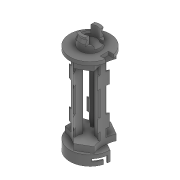
# Autodesk Inventor part: Sujección_Baterias
Saved by Autodesk Inventor 2022.3 (Build 263350000, 350)
## iProperties
Created: 2023-07-18
Part Number: Sujección_Baterias
Material: Genérico
Document SubType Name: Modeling
Designer: Usuario
Density: 1 g/cm^3
Appearance: Valor por defecto
Author: Usuario
Autodesk Inventor part; units mm, degrees
ref_plane "YZ Plane" through (0, 0, 0) normal (1, 0, 0) x (0, 1, 0)
ref_plane "XZ Plane" through (0, 0, 0) normal (0, 1, 0) x (-1, 0, 0)
ref_plane "XY Plane" through (0, 0, 0) normal (0, 0, 1) x (1, 0, 0)
sketch "Boceto1" plane through (0, 0, 0) normal (0, 1, 0) x (-1, 0, 0)
  circle A0 centre (0, 0) radius 10.5
  circle A1 centre (0, 0) radius 7.25
  dimension "d0" = 21
  dimension "d1" = 14.5
  constraints: 2 centre point, 2 coincident
  measures "d0" diameter of A0
  measures "d1" diameter of A1
extrude "Extrusión1" add sketch "Boceto1" along normal blind 14
sketch "Boceto2" plane through (0, 14, 0) normal (0, 1, 0) x (1, 0, 0)
  line L0 (0, 0) -> (-4.6, 0)
  line L1 (-4.6, 0) -> (-4.6, -9.4387)
  circle A0 centre (0, 0) radius 10.5 projected
  line L2 (-4.6, 0) -> (-4.6, 9.4387)
  line L3 (0, 0) -> (4.6, 0)
  line L4 (4.6, 0) -> (4.6, -9.4387)
  line L5 (4.6, 0) -> (4.6, 9.4387)
  circle A1 centre (0, 0) radius 10.5
  dimension "d4" = 4.6
  dimension "d5" = 4.6
  constraints: 12 end point, 4 point on circle, 3 point on line, 2 perpendicular, 1 centre point, 1 coincident, 1 horizontal
  measures "d4" distance of L0.start L0.end
  measures "d5" distance of L3.start L3.end
extrude "Extrusión2" cut sketch "Boceto2" against normal blind 8 contours L1 A0 L2 | L5 A0 L4
sketch "Boceto3" plane through (0, 6, 0) normal (0, 1, 0) x (1, 0, 0)
  arc A0 (4.6, -9.4387) -> (4.6, 9.4387) centre (0, 0) ccw projected
  line L0 (10.5, 0) -> (7.25, 0)
  circle A1 centre (0, 0) radius 7.25 projected
  line L1 (8.875, 0) -> (8.875, -5)
  line L2 (8.875, -5) -> (5.25, -5)
  line L3 (8.875, 0) -> (8.875, 5)
  line L4 (8.875, 5) -> (5.25, 5)
  line L5 (8.875, -5) -> (9.2331, -5)
  line L6 (8.875, 5) -> (9.2331, 5)
  arc A2 (4.6, -5.6038) -> (4.6, 5.6038) centre (0, 0) ccw projected
  dimension "d8" = 5
  dimension "d9" = 5
  constraints: 14 end point, 6 point on circle, 3 perpendicular, 2 vertical, 1 horizontal, 1 midpoint, 1 parallel
  measures "d8" distance of L1.start L1.end
  measures "d9" distance of L1.start L3.end
extrude "Extrusión3" cut sketch "Boceto3" against normal blind 3 contours L5 L1 L0 A0 | L0 L3 L6 A0 | L2 A1 L0 L1 | L0 A1 L4 L3
sketch "Boceto4" plane through (0, 0, 0) normal (1, 0, 0) x (0, 1, 0)
  line L0 (14, 9.4387) -> (14, 10.5) projected
  line L1 (14, 5.6038) -> (6, 5.6038) projected
  line L2 (7.5, 8.75) -> (14, 8.75)
  line L3 (14, 12.25) -> (7.5, 12.25)
  line L4 (7.5, 12.25) -> (7.5, 8.75)
  line L5 (7.5, 10.5) -> (10.75, 8.75)
  line L6 (10.75, 8.75) -> (14, 10.5)
  line L7 (14, 10.5) -> (14, 12.25)
  line L8 (14, 10.5) -> (14, 8.75)
  line L9 (14, 8.75) -> (7.5, 8.75)
  line L10 (7.5, 8.75) -> (7.5, 10.5)
  point P0 (0, 0)
  constraints: 18 end point, 3 perpendicular, 2 midpoint, 1 parallel
sketch3d "Boceto 3D1"
  arc A0 (-10.5, 0, 0) -> (0, 0, 10.5) centre (0, 0, 0) ccw
  arc A1 (0, 0, 10.5) -> (10.5, 0, 0) centre (0, 0, 0) ccw
  arc A2 (10.5, 0, 0) -> (0, 0, -10.5) centre (0, 0, 0) ccw
  arc A3 (0, 0, -10.5) -> (-10.5, 0, 0) centre (0, 0, 0) ccw
sweep "Barrido1" cut profiles "Boceto4" path "Boceto 3D1" contours L6 L5 L4 L3 L7
sketch "Boceto6" plane through (0, 3, 0) normal (0, 1, 0) x (1, 0, 0)
  circle A0 centre (0, 0) radius 7.25
  constraints: 1 centre point, 1 coincident
extrude "Extrusión4" add sketch "Boceto6" against normal blind 3
sketch "Boceto5" plane through (0, 0, 0) normal (0, -1, 0) x (1, 0, 0)
  circle A0 centre (0, 0) radius 21
  dimension "d16" = 42
  constraints: 1 centre point, 1 coincident
  measures "d16" diameter of A0
extrude "Extrusión5" add sketch "Boceto5" along normal blind 3.7
sketch "Boceto7" plane through (0, -3.7, 0) normal (0, -1, 0) x (1, 0, 0)
  circle A0 centre (0, 0) radius 21 projected
  line L0 (-21, 0) -> (15, 0)
  line L1 (15, 0) -> (15, 4.375)
  line L2 (15, 4.375) -> (20.5392, 4.375)
  line L3 (15, 0) -> (15, -4.375)
  line L4 (15, -4.375) -> (20.5392, -4.375)
  circle A1 centre (0, 0) radius 21 projected
  dimension "d19" = 36
  dimension "d20" = 4.375
  dimension "d21" = 4.375
  constraints: 10 end point, 3 point on circle, 1 horizontal, 1 perpendicular, 1 point on line, 1 vertical
  measures "d19" distance of L0.start L0.end
  measures "d20" distance of L0.end L1.end
  measures "d21" distance of L0.end L3.end
extrude "Extrusión6" cut sketch "Boceto7" against normal through all contours A0 L4 L3 L1 L2
sketch "Boceto8" plane through (0, -3.7, 0) normal (0, -1, 0) x (1, 0, 0)
  arc A0 (4.6, 9.4387) -> (-4.6, 9.4387) centre (0, 0) ccw projected
  arc A1 (20.5392, 4.375) -> (20.5392, -4.375) centre (0, 0) ccw projected
  line L0 (-21, 0) -> (10.5, 18.1865)
  line L1 (10.5, 18.1865) -> (10.5, -18.1865)
  line L2 (10.5, -18.1865) -> (-21, 0)
  line L3 (10.5, 18.1865) -> (0, 0)
  line L4 (0, 0) -> (10.5, -18.1865)
  line L5 (0, 0) -> (-21, 0)
  line L6 (10.5, 18.1865) -> (6, 10.3923)
  line L7 (10.5, -18.1865) -> (6, -10.3923)
  line L8 (-21, 0) -> (-12, 0)
  circle A2 centre (-12, 0) radius 9
  circle A3 centre (6, -10.3923) radius 9
  circle A4 centre (6, 10.3923) radius 9
  line L9 (0, 0) -> (-22.5, 38.9711)
  circle A5 centre (-22.5, 38.9711) radius 31.3609
  line L10 (0, 0) -> (-22.5, -38.9711)
  line L11 (0, 0) -> (45, 0)
  circle A6 centre (-22.5, -38.9711) radius 31.3609
  circle A7 centre (45, 0) radius 31.3609
  line L12 (10.5, 18.1865) -> (9, 15.5885)
  line L13 (9, 15.5885) -> (2.1283, 19.5559)
  line L14 (9, 15.5885) -> (15.8717, 11.6211)
  line L15 (-21, 0) -> (-18, 0)
  line L16 (-18, 0) -> (-18, 7.9348)
  line L17 (-18, 0) -> (-18, -7.9348)
  line L18 (10.5, -18.1865) -> (9, -15.5885)
  line L19 (9, -15.5885) -> (15.8717, -11.6211)
  line L20 (9, -15.5885) -> (2.1283, -19.5559)
  dimension "d24" = 9
  dimension "d25" = 9
  dimension "d26" = 45
  dimension "d27" = 45
  dimension "d28" = 45
  dimension "d29" = 3
  dimension "d30" = 3
  dimension "d31" = 3
  constraints: 42 end point, 8 point on line, 7 coincident, 7 point on circle, 3 centre point, 3 perpendicular, 2 horizontal, 1 horizontal alignment, 18 other
  measures "d24" distance of L0.end L6.end
  measures "d25" distance of L0.start L8.end
  measures "d26" distance of L3.end L9.end
  measures "d27" distance of L3.end L10.end
  measures "d28" distance of L3.end L11.end
  measures "d29" distance of L0.end L12.end
  measures "d30" distance of L0.start L15.end
  measures "d31" distance of L1.end L18.end
extrude "Extrusión7" add sketch "Boceto8" along normal blind 6.3 contours A7 A4 L14 | L13 L3 A4 L0 | L0 A4 L13 | L14 A4 L1 | L1 A4 L3 L14 | A4 A5 L13 | A7 L11 L1 A4 | A4 L3 L9 L0 | L0 L9 A5 A4 | L1 L11 L3 A4 | L19 A3 A7 | A7 A3 L1 L11 | L9 L0 A2 A5 | L9 L5 A2 L0 | L1 A3 L4 L11 | L19 L4 A3 L1 | L1 A3 L19 | L20 A3 L2 | L2 A3 L4 L20 | L20 A6 A3 | A5 A2 L16 | A2 L0 L16 | A2 L5 L16 L0 | L10 L2 A2 L5 | L4 A3 L2 L10 | A3 A6 L10 L2 | L17 L5 A2 L2 | L2 A2 L17 | A2 A6 L17 | L10 A6 A2 L2 picked at (0.5579, 12.9993) picked at (10.9788, 6.9828) picked at (10.9788, -6.9828) picked at (0.5579, -12.9993) picked at (-11.5367, 6.0165) picked at (-11.5367, -6.0165)
sketch "Boceto9" plane through (0, -10, 0) normal (0, -1, 0) x (1, 0, 0)
  arc A0 (4.6, 9.4387) -> (-4.6, 9.4387) centre (0, 0) ccw
  arc A1 (20.5392, 4.375) -> (20.5392, -4.375) centre (0, 0) ccw
  line L0 (-21, 0) -> (10.5, 18.1865)
  line L1 (10.5, 18.1865) -> (10.5, -18.1865)
  line L2 (10.5, -18.1865) -> (-21, 0)
  line L3 (10.5, 18.1865) -> (0, 0)
  line L4 (0, 0) -> (10.5, -18.1865)
  line L5 (0, 0) -> (-21, 0)
  line L6 (10.5, 18.1865) -> (6, 10.3923)
  line L7 (10.5, -18.1865) -> (6, -10.3923)
  line L8 (-21, 0) -> (-12, 0)
  circle A2 centre (-12, 0) radius 9
  circle A3 centre (6, -10.3923) radius 9
  circle A4 centre (6, 10.3923) radius 9
  line L9 (0, 0) -> (-22.5, 38.9711)
  circle A5 centre (-22.5, 38.9711) radius 31.3609
  line L10 (0, 0) -> (-22.5, -38.9711)
  line L11 (0, 0) -> (45, 0)
  circle A6 centre (-22.5, -38.9711) radius 31.3609
  circle A7 centre (45, 0) radius 31.3609
  line L12 (10.5, 18.1865) -> (9, 15.5885)
  line L13 (9, 15.5885) -> (2.1283, 19.5559)
  line L14 (9, 15.5885) -> (15.8717, 11.6211)
  line L15 (-21, 0) -> (-18, 0)
  line L16 (-18, 0) -> (-18, 7.9348)
  line L17 (-18, 0) -> (-18, -7.9348)
  line L18 (10.5, -18.1865) -> (9, -15.5885)
  line L19 (9, -15.5885) -> (15.8717, -11.6211)
  line L20 (9, -15.5885) -> (2.1283, -19.5559)
  line L21 (6, 10.3923) -> (-12, 0)
  line L22 (-12, 0) -> (6, -10.3923)
  line L23 (6, -10.3923) -> (6, 10.3923)
  point P0 (-1.7942, -5.8923)
  point P1 (-4.2058, -4.5)
  point P2 (-14.3414, -8.6901)
  point P3 (-0.3552, -16.765)
  point P4 (-0.3552, 16.765)
  point P5 (-14.3414, 8.6901)
  point P6 (-4.2058, 4.5)
  point P7 (-1.7942, 5.8923)
  point P8 (14.6965, -8.0749)
  point P9 (14.6965, 8.0749)
  point P10 (6, 1.3923)
  point P11 (6, -1.3923)
  dimension "d34" = 9
  dimension "d35" = 9
  dimension "d36" = 45
  dimension "d37" = 45
  dimension "d38" = 45
  dimension "d39" = 3
  dimension "d40" = 3
  dimension "d41" = 3
  constraints: 48 end point, 11 point on circle, 9 point on line, 7 coincident, 5 centre point, 3 perpendicular, 2 horizontal, 1 vertical, 19 other
  measures "d34" distance of L0.end L6.end
  measures "d35" distance of L0.start L8.end
  measures "d36" distance of L3.end L9.end
  measures "d37" distance of L3.end L10.end
  measures "d38" distance of L3.end L11.end
  measures "d39" distance of L0.end L12.end
  measures "d40" distance of L0.start L15.end
  measures "d41" distance of L1.end L18.end
extrude "Extrusión8" add sketch "Boceto9" along normal blind 68.25 contours A4 L21 L9 L0 | L0 L9 A5 A4 | A4 L1 L11 L23 | L21 A2 L0 L9 | L0 A2 A5 L9 | A4 A7 L11 L1 | L11 L1 A3 L23 | L22 A3 L2 L10 | L10 L2 A2 L22 | L11 A7 A3 L1 | L10 A6 A2 L2 | L2 A3 A6 L10
fillet "Empalme1" radius 1 6 edges at (-14.3414, -44.125, 8.6901) (-0.3552, -44.125, 16.765) (-14.3414, -44.125, -8.6901) (14.6965, -44.125, -8.0749) (14.6965, -44.125, 8.0749) (-0.3552, -44.125, -16.765)
ref_plane "Plano de trabajo1" through (0, -18.35, 0) normal (0, -1, 0) x (1, 0, 0)
sketch "Boceto10" plane through (0, -18.35, 0) normal (0, -1, 0) x (1, 0, 0)
  arc A0 (4.6, 9.4387) -> (-4.6, 9.4387) centre (0, 0) ccw
  arc A1 (20.5392, 4.375) -> (20.5392, -4.375) centre (0, 0) ccw
  line L0 (-21, 0) -> (10.5, 18.1865)
  line L1 (10.5, 18.1865) -> (10.5, -18.1865)
  line L2 (10.5, -18.1865) -> (-21, 0)
  line L3 (10.5, 18.1865) -> (0, 0)
  line L4 (0, 0) -> (10.5, -18.1865)
  line L5 (0, 0) -> (-21, 0)
  line L6 (10.5, 18.1865) -> (6, 10.3923)
  line L7 (10.5, -18.1865) -> (6, -10.3923)
  line L8 (-21, 0) -> (-12, 0)
  circle A2 centre (-12, 0) radius 9
  circle A3 centre (6, -10.3923) radius 9
  circle A4 centre (6, 10.3923) radius 9
  line L9 (0, 0) -> (-22.5, 38.9711)
  circle A5 centre (-22.5, 38.9711) radius 31.3609
  line L10 (0, 0) -> (-22.5, -38.9711)
  line L11 (0, 0) -> (45, 0)
  circle A6 centre (-22.5, -38.9711) radius 31.3609
  circle A7 centre (45, 0) radius 31.3609
  line L12 (10.5, 18.1865) -> (9, 15.5885)
  line L13 (9, 15.5885) -> (2.1283, 19.5559)
  line L14 (9, 15.5885) -> (15.8717, 11.6211)
  line L15 (-21, 0) -> (-18, 0)
  line L16 (-18, 0) -> (-18, 7.9348)
  line L17 (-18, 0) -> (-18, -7.9348)
  line L18 (10.5, -18.1865) -> (9, -15.5885)
  line L19 (9, -15.5885) -> (15.8717, -11.6211)
  line L20 (9, -15.5885) -> (2.1283, -19.5559)
  line L21 (6, 10.3923) -> (-12, 0)
  line L22 (-12, 0) -> (6, -10.3923)
  line L23 (6, -10.3923) -> (6, 10.3923)
  point P0 (-1.7942, -5.8923)
  point P1 (-4.2058, -4.5)
  point P2 (-14.3414, -8.6901)
  point P3 (-0.3552, -16.765)
  point P4 (-0.3552, 16.765)
  point P5 (-14.3414, 8.6901)
  point P6 (-4.2058, 4.5)
  point P7 (-1.7942, 5.8923)
  point P8 (14.6965, -8.0749)
  point P9 (14.6965, 8.0749)
  point P10 (6, 1.3923)
  point P11 (6, -1.3923)
  point P12 (14.6965, 8.0749)
  point P13 (10.5, 2.5981)
  point P14 (10.5, -2.5981)
  point P15 (14.6965, -8.0749)
  point P16 (-14.3414, -8.6901)
  point P17 (-0.3552, -16.765)
  point P18 (-3, -10.3923)
  point P19 (-7.5, -7.7942)
  point P20 (-14.3414, 8.6901)
  point P21 (-7.5, 7.7942)
  point P22 (-3, 10.3923)
  point P23 (-0.3552, 16.765)
  dimension "d46" = 9
  dimension "d47" = 9
  dimension "d48" = 45
  dimension "d49" = 45
  dimension "d50" = 45
  dimension "d51" = 3
  dimension "d52" = 3
  dimension "d53" = 3
  constraints: 48 end point, 11 point on circle, 9 point on line, 7 coincident, 5 centre point, 3 perpendicular, 2 horizontal, 1 vertical, 19 other
  measures "d46" distance of L0.end L6.end
  measures "d47" distance of L0.start L8.end
  measures "d48" distance of L3.end L9.end
  measures "d49" distance of L3.end L10.end
  measures "d50" distance of L3.end L11.end
  measures "d51" distance of L0.end L12.end
  measures "d52" distance of L0.start L15.end
  measures "d53" distance of L1.end L18.end
extrude "Extrusión9" add sketch "Boceto10" along normal blind 12.75 contours L0 L9 A5 A4 | L0 A2 A5 L9 | A4 A7 L11 L1 | L11 A7 A3 L1 | L10 A6 A2 L2 | L2 A3 A6 L10
ref_plane "Plano de trabajo2" through (0, -57.25, 0) normal (0, -1, 0) x (1, 0, 0)
sketch "Boceto11" plane through (0, -57.25, 0) normal (0, -1, 0) x (1, 0, 0)
  arc A0 (4.6, 9.4387) -> (-4.6, 9.4387) centre (0, 0) ccw
  arc A1 (20.5392, 4.375) -> (20.5392, -4.375) centre (0, 0) ccw
  line L0 (-21, 0) -> (10.5, 18.1865)
  line L1 (10.5, 18.1865) -> (10.5, -18.1865)
  line L2 (10.5, -18.1865) -> (-21, 0)
  line L3 (10.5, 18.1865) -> (0, 0)
  line L4 (0, 0) -> (10.5, -18.1865)
  line L5 (0, 0) -> (-21, 0)
  line L6 (10.5, 18.1865) -> (6, 10.3923)
  line L7 (10.5, -18.1865) -> (6, -10.3923)
  line L8 (-21, 0) -> (-12, 0)
  circle A2 centre (-12, 0) radius 9
  circle A3 centre (6, -10.3923) radius 9
  circle A4 centre (6, 10.3923) radius 9
  line L9 (0, 0) -> (-22.5, 38.9711)
  circle A5 centre (-22.5, 38.9711) radius 31.3609
  line L10 (0, 0) -> (-22.5, -38.9711)
  line L11 (0, 0) -> (45, 0)
  circle A6 centre (-22.5, -38.9711) radius 31.3609
  circle A7 centre (45, 0) radius 31.3609
  line L12 (10.5, 18.1865) -> (9, 15.5885)
  line L13 (9, 15.5885) -> (2.1283, 19.5559)
  line L14 (9, 15.5885) -> (15.8717, 11.6211)
  line L15 (-21, 0) -> (-18, 0)
  line L16 (-18, 0) -> (-18, 7.9348)
  line L17 (-18, 0) -> (-18, -7.9348)
  line L18 (10.5, -18.1865) -> (9, -15.5885)
  line L19 (9, -15.5885) -> (15.8717, -11.6211)
  line L20 (9, -15.5885) -> (2.1283, -19.5559)
  line L21 (6, 10.3923) -> (-12, 0)
  line L22 (-12, 0) -> (6, -10.3923)
  line L23 (6, -10.3923) -> (6, 10.3923)
  point P0 (-1.7942, -5.8923)
  point P1 (-4.2058, -4.5)
  point P2 (-14.3414, -8.6901)
  point P3 (-0.3552, -16.765)
  point P4 (-0.3552, 16.765)
  point P5 (-14.3414, 8.6901)
  point P6 (-4.2058, 4.5)
  point P7 (-1.7942, 5.8923)
  point P8 (14.6965, -8.0749)
  point P9 (14.6965, 8.0749)
  point P10 (6, 1.3923)
  point P11 (6, -1.3923)
  point P12 (14.6965, -8.0749)
  point P13 (14.6965, 8.0749)
  point P14 (10.5, 2.5981)
  point P15 (10.5, -2.5981)
  point P16 (-14.3414, -8.6901)
  point P17 (-0.3552, -16.765)
  point P18 (-3, -10.3923)
  point P19 (-7.5, -7.7942)
  point P20 (-14.3414, 8.6901)
  point P21 (-7.5, 7.7942)
  point P22 (-3, 10.3923)
  point P23 (-0.3552, 16.765)
  dimension "d57" = 9
  dimension "d58" = 9
  dimension "d59" = 45
  dimension "d60" = 45
  dimension "d61" = 45
  dimension "d62" = 3
  dimension "d63" = 3
  dimension "d64" = 3
  constraints: 48 end point, 11 point on circle, 9 point on line, 7 coincident, 5 centre point, 3 perpendicular, 2 horizontal, 1 vertical, 19 other
  measures "d57" distance of L0.end L6.end
  measures "d58" distance of L0.start L8.end
  measures "d59" distance of L3.end L9.end
  measures "d60" distance of L3.end L10.end
  measures "d61" distance of L3.end L11.end
  measures "d62" distance of L0.end L12.end
  measures "d63" distance of L0.start L15.end
  measures "d64" distance of L1.end L18.end
extrude "Extrusión10" add sketch "Boceto11" along normal blind 12.75 contours L0 L9 A5 A4 | L0 A2 A5 L9 | A4 A7 L11 L1 | L11 A7 A3 L1 | L10 A6 A2 L2 | L2 A3 A6 L10
sketch "Boceto13" plane through (0, -78.25, 0) normal (0, -1, 0) x (1, 0, 0)
  line L0 (15.8717, -11.6211) -> (2.1283, -19.5559)
  arc A0 (2.1283, -19.5559) -> (-18, -7.9348) centre (-22.5, -38.9711) ccw
  line L1 (-18, -7.9348) -> (-18, 7.9348)
  arc A1 (-18, 7.9348) -> (2.1283, 19.5559) centre (-22.5, 38.9711) ccw
  line L2 (2.1283, 19.5559) -> (15.8717, 11.6211)
  arc A2 (15.8717, 11.6211) -> (15.8717, -11.6211) centre (45, 0) ccw
  point P0 (0, 0)
  point P1 (0, 0)
  constraints: 6 end point, 6 point on circle, 3 centre point
extrude "Extrusión11" add sketch "Boceto13" along normal blind 6.3
sketch "Boceto14" plane through (0, -84.55, 0) normal (0, -1, 0) x (1, 0, 0)
  circle A0 centre (0, 0) radius 21
  arc A1 (2.1283, -19.5559) -> (-18, -7.9348) centre (-22.5, -38.9711) ccw projected
  line L0 (0, 0) -> (-22.5, -38.9711)
  line L1 (21, 0) -> (-10.5, -18.1865)
  arc A2 (20.5392, 4.375) -> (20.5392, -4.375) centre (0, 0) ccw projected
  point P0 (-3.4076, -14.0917)
  point P1 (-10.5, -18.1865)
  point P2 (-6.8196, -11.8118)
  constraints: 4 end point, 2 point on circle, 1 centre point, 1 coincident, 1 point on line
extrude "Extrusión12" add sketch "Boceto14" along normal blind 10.5 contours L1 A1 L0 A0 | L1 L0 A1
sketch "Boceto15" plane through (0, -95.05, 0) normal (0, -1, 0) x (1, 0, 0)
  arc A0 (5.25, 5) -> (5.25, -5) centre (0, 0) ccw projected
  circle A1 centre (0, 0) radius 21
  circle A2 centre (0, 0) radius 20
  arc A3 (21, 0) -> (-10.5, -18.1865) centre (0, 0) ccw projected
  line L0 (21, 0) -> (19.9915, -0.5822)
  line L1 (-10.5, -18.1865) -> (21, 0) projected
  line L2 (-10.5, -18.1865) -> (1.6244, -11.1865)
  line L3 (1.6244, -11.1865) -> (1.1244, -10.3205)
  line L4 (1.1244, -10.3205) -> (-10.4918, -17.0271)
  line L5 (1.6244, -11.1865) -> (19.9915, -0.5822)
  dimension "d71" = 40
  dimension "d72" = 14
  dimension "d73" = 1
  constraints: 10 end point, 3 point on circle, 3 point on line, 2 centre point, 2 coincident, 2 perpendicular, 1 parallel
  measures "d71" diameter of A2
  measures "d72" distance of L2.start L2.end
  measures "d73" distance of L2.end L3.end
extrude "Extrusión13" cut sketch "Boceto15" against normal blind 6.8 contours L1 L3 L4 A2 picked at (0.1121, 9.7909)
fillet "Empalme2" radius 0.15 10 edges at (-0.3552, -63.625, -16.765) (14.6965, -63.625, -8.0749) (14.6965, -24.725, -8.0749) (-0.3552, -24.725, -16.765) (-14.3414, -24.725, -8.6901) (-14.3414, -63.625, -8.6901) (14.6965, -63.625, 8.0749) (14.6965, -24.725, 8.0749) (-14.3414, -24.725, 8.6901) (-14.3414, -63.625, 8.6901)
sketch "Boceto16" plane through (-10.5, -95.05, -18.1865) normal (0.5, 0, -0.8660254) x (-0.8660254, 0, -0.5)
  line L0 (-14, 0) -> (-14, 6.8) projected
  line L1 (-14, 3.4) -> (0, 3.4)
  line L2 (0, 10.5) -> (0, 0) projected
  circle A0 centre (-7, 3.4) radius 1.5
  point P0 (-18.1865, 95.05)
  dimension "d77" = 3
  constraints: 2 end point, 2 midpoint, 1 centre point, 1 horizontal, 1 point on line
  measures "d77" diameter of A0
extrude "Extrusión14" cut sketch "Boceto16" against normal up to surface (1 mm away)
sketch "Boceto17" plane through (0, -95.05, 0) normal (0, -1, 0) x (1, 0, 0)
  arc A0 (21, 0) -> (-10.5, -18.1865) centre (0, 0) ccw projected
  arc A1 (19.9915, -0.5822) -> (-10.4918, -17.0271) centre (0, 0) ccw projected
  arc A2 (19.9915, -0.5822) -> (-10.4918, -17.0271) centre (0, 0) ccw projected
  line L0 (19.9915, -0.5822) -> (19.8537, 2.4146)
  line L1 (19.8537, 2.4146) -> (20.8464, 2.5353)
  line L2 (19.8537, 2.4146) -> (19.1288, 5.8387)
  line L3 (19.1288, 5.8387) -> (20.1107, 6.0466)
  line L4 (-10.5, -18.1865) -> (-3.4076, -14.0917) projected
  line L5 (-10.5, -18.1865) -> (-19.6914, -7.2971)
  arc A3 (20.5392, 4.375) -> (20.5392, -4.375) centre (0, 0) ccw projected
  line L6 (-19.6914, -7.2971) -> (-18.8764, -6.6092)
  line L7 (-19.6914, -7.2971) -> (-20.7178, -3.431)
  line L8 (-20.7178, -3.431) -> (-19.8205, -2.6736)
  dimension "d80" = 3
  dimension "d81" = 1
  dimension "d82" = 3.5
  dimension "d89" = 14.25
  dimension "d90" = 4
  constraints: 16 end point, 8 point on circle, 2 perpendicular
  measures "d80" distance of L0.start L0.end
  measures "d81" distance of L0.end L1.end
  measures "d82" distance of L0.end L2.end
  measures "d89" distance of L4.start L5.end
  measures "d90" distance of L5.end L7.end
extrude "Extrusión15" cut sketch "Boceto17" against normal up to surface (6.8 mm away) contours L1 A1 L3 A0 | L2 A1 | L7 A0 | L8 A1 L6 L7
sketch "Boceto18" plane through (0, -88.25, 0) normal (0, -1, 0) x (1, 0, 0)
  line L0 (19.1288, 5.8387) -> (20.1107, 6.0466) projected
  arc A0 (20.1107, 6.0466) -> (-20.7178, -3.431) centre (0, 0) ccw projected
  line L1 (-10.5, -18.1865) -> (1.6244, -11.1865) projected
  line L2 (1.6244, -11.1865) -> (1.1244, -10.3205) projected
  line L3 (1.1244, -10.3205) -> (-10.4918, -17.0271) projected
  arc A1 (19.9915, -0.5822) -> (19.8537, 2.4146) centre (0, 0) ccw projected
  arc A2 (19.1288, 5.8387) -> (-10.4918, -17.0271) centre (0, 0) ccw projected
  line L4 (19.1288, 5.8387) -> (14.6319, 13.6347)
  line L5 (20.1107, 6.0466) -> (15.7326, 13.9099)
  arc A3 (21, 0) -> (-10.5, -18.1865) centre (0, 0) ccw projected
  line L6 (15.7326, 13.9099) -> (14.6319, 13.6347)
  line L7 (20.8464, 2.5353) -> (19.8537, 2.4146) projected
  line L8 (19.9915, -0.5822) -> (21, 0) projected
  arc A4 (21, 0) -> (20.8464, 2.5353) centre (0, 0) ccw projected
  line L9 (-20.7178, -3.431) -> (-19.8205, -2.6736) projected
  arc A5 (19.1288, 5.8387) -> (-19.8205, -2.6736) centre (0, 0) ccw projected
  line L10 (-18.8764, -6.6092) -> (-19.6914, -7.2971) projected
  arc A6 (-19.6914, -7.2971) -> (-10.5, -18.1865) centre (0, 0) ccw projected
  arc A7 (-18.8764, -6.6092) -> (-10.4918, -17.0271) centre (0, 0) ccw projected
  line L11 (-18.8764, -6.6092) -> (-19.6914, -7.2971) projected
  line L12 (-18.8764, -6.6092) -> (-14.0673, -14.2166)
  line L13 (-14.0673, -14.2166) -> (-14.9337, -14.7643)
  arc A8 (20.5392, 4.375) -> (20.5392, -4.375) centre (0, 0) ccw projected
  dimension "d85" = 9
  dimension "d86" = 9
  dimension "d91" = 9
  constraints: 10 end point, 3 point on circle
  measures "d85" distance of L0.start L4.end
  measures "d86" distance of L0.end L5.end
  measures "d91" distance of L10.start L12.end
extrude "Extrusión16" cut sketch "Boceto18" along normal blind 2.5 contours A2 L6 L5 L0 | L5 A0 | L12 A2 | A2 L13 A3 L10
